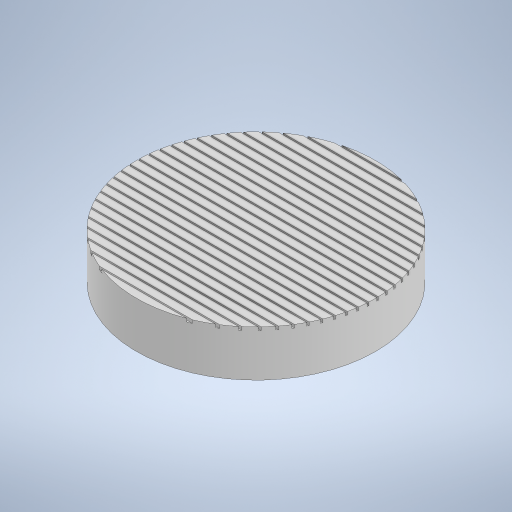
# Autodesk Inventor part: CircularTeflonHolder
Saved by Autodesk Inventor 2024 (Build 280153000, 153)
## iProperties
Created: 2023-08-11
Part Number: CircularTeflonHolder
Material: Generic
Document SubType Name: Modeling
Designer: Edwin
Density: 1 g/cm^3
Appearance: Default
Author: Edwin
Autodesk Inventor part; units mm, degrees
ref_plane "YZ Plane" through (0, 0, 0) normal (1, 0, 0) x (0, 1, 0)
ref_plane "XZ Plane" through (0, 0, 0) normal (0, 1, 0) x (-1, 0, 0)
ref_plane "XY Plane" through (0, 0, 0) normal (0, 0, 1) x (1, 0, 0)
sketch "Sketch1" plane through (0, 0, 0) normal (0, 1, 0) x (-1, 0, 0)
  circle A0 centre (0, 0) radius 38.1
  dimension "d0" = 76.2
  constraints: 1 centre point, 1 coincident
  measures "d0" diameter of A0
extrude "Extrusion1" add sketch "Sketch1" along normal blind 12.7
sketch "Sketch2" plane through (0, 0, 0) normal (0, -1, 0) x (1, 0, 0)
  circle A0 centre (0, 0) radius 38.1 projected
  circle A1 centre (0, 0) radius 32.1
  dimension "d3" = 6
  constraints: 1 centre point, 1 coincident
  measures "d3" radial gap between concentric circles of A0 A1
extrude "Extrusion2" add sketch "Sketch2" along normal blind 2
sketch "Sketch3" plane through (0, 0, 0) normal (1, 0, 0) x (0, 1, 0)
  line L0 (12.7, -38.1) -> (12.7, 38.1) projected
  line L1 (12.7, 38.1) -> (11.7, 38.1)
  line L2 (11.7, 38.1) -> (11.7, 38.6)
  line L3 (11.7, 38.6) -> (12.7, 38.6)
  line L4 (12.7, 38.6) -> (12.7, 38.1)
  line L5 (12.7, 35.1) -> (11.7, 35.1)
  line L6 (11.7, 35.1) -> (11.7, 35.6)
  line L7 (11.7, 35.6) -> (12.7, 35.6)
  line L8 (12.7, 35.6) -> (12.7, 35.1)
  line L9 (12.7, 32.1) -> (11.7, 32.1)
  line L10 (11.7, 32.1) -> (11.7, 32.6)
  line L11 (11.7, 32.6) -> (12.7, 32.6)
  line L12 (12.7, 32.6) -> (12.7, 32.1)
  line L13 (12.7, 29.1) -> (11.7, 29.1)
  line L14 (11.7, 29.1) -> (11.7, 29.6)
  line L15 (11.7, 29.6) -> (12.7, 29.6)
  line L16 (12.7, 29.6) -> (12.7, 29.1)
  line L17 (12.7, 26.1) -> (11.7, 26.1)
  line L18 (11.7, 26.1) -> (11.7, 26.6)
  line L19 (11.7, 26.6) -> (12.7, 26.6)
  line L20 (12.7, 26.6) -> (12.7, 26.1)
  line L21 (12.7, 23.1) -> (11.7, 23.1)
  line L22 (11.7, 23.1) -> (11.7, 23.6)
  line L23 (11.7, 23.6) -> (12.7, 23.6)
  line L24 (12.7, 23.6) -> (12.7, 23.1)
  line L25 (12.7, 20.1) -> (11.7, 20.1)
  line L26 (11.7, 20.1) -> (11.7, 20.6)
  line L27 (11.7, 20.6) -> (12.7, 20.6)
  line L28 (12.7, 20.6) -> (12.7, 20.1)
  line L29 (12.7, 17.1) -> (11.7, 17.1)
  line L30 (11.7, 17.1) -> (11.7, 17.6)
  line L31 (11.7, 17.6) -> (12.7, 17.6)
  line L32 (12.7, 17.6) -> (12.7, 17.1)
  line L33 (12.7, 14.1) -> (11.7, 14.1)
  line L34 (11.7, 14.1) -> (11.7, 14.6)
  line L35 (11.7, 14.6) -> (12.7, 14.6)
  line L36 (12.7, 14.6) -> (12.7, 14.1)
  line L37 (12.7, 11.1) -> (11.7, 11.1)
  line L38 (11.7, 11.1) -> (11.7, 11.6)
  line L39 (11.7, 11.6) -> (12.7, 11.6)
  line L40 (12.7, 11.6) -> (12.7, 11.1)
  line L41 (12.7, 8.1) -> (11.7, 8.1)
  line L42 (11.7, 8.1) -> (11.7, 8.6)
  line L43 (11.7, 8.6) -> (12.7, 8.6)
  line L44 (12.7, 8.6) -> (12.7, 8.1)
  line L45 (12.7, 5.1) -> (11.7, 5.1)
  line L46 (11.7, 5.1) -> (11.7, 5.6)
  line L47 (11.7, 5.6) -> (12.7, 5.6)
  line L48 (12.7, 5.6) -> (12.7, 5.1)
  line L49 (12.7, 2.1) -> (11.7, 2.1)
  line L50 (11.7, 2.1) -> (11.7, 2.6)
  line L51 (11.7, 2.6) -> (12.7, 2.6)
  line L52 (12.7, 2.6) -> (12.7, 2.1)
  line L53 (12.7, -0.9) -> (11.7, -0.9)
  line L54 (11.7, -0.9) -> (11.7, -0.4)
  line L55 (11.7, -0.4) -> (12.7, -0.4)
  line L56 (12.7, -0.4) -> (12.7, -0.9)
  line L57 (12.7, -3.9) -> (11.7, -3.9)
  line L58 (11.7, -3.9) -> (11.7, -3.4)
  line L59 (11.7, -3.4) -> (12.7, -3.4)
  line L60 (12.7, -3.4) -> (12.7, -3.9)
  line L61 (12.7, -6.9) -> (11.7, -6.9)
  line L62 (11.7, -6.9) -> (11.7, -6.4)
  line L63 (11.7, -6.4) -> (12.7, -6.4)
  line L64 (12.7, -6.4) -> (12.7, -6.9)
  line L65 (12.7, -9.9) -> (11.7, -9.9)
  line L66 (11.7, -9.9) -> (11.7, -9.4)
  line L67 (11.7, -9.4) -> (12.7, -9.4)
  line L68 (12.7, -9.4) -> (12.7, -9.9)
  line L69 (12.7, -12.9) -> (11.7, -12.9)
  line L70 (11.7, -12.9) -> (11.7, -12.4)
  line L71 (11.7, -12.4) -> (12.7, -12.4)
  line L72 (12.7, -12.4) -> (12.7, -12.9)
  line L73 (12.7, -15.9) -> (11.7, -15.9)
  line L74 (11.7, -15.9) -> (11.7, -15.4)
  line L75 (11.7, -15.4) -> (12.7, -15.4)
  line L76 (12.7, -15.4) -> (12.7, -15.9)
  line L77 (12.7, -18.9) -> (11.7, -18.9)
  line L78 (11.7, -18.9) -> (11.7, -18.4)
  line L79 (11.7, -18.4) -> (12.7, -18.4)
  line L80 (12.7, -18.4) -> (12.7, -18.9)
  line L81 (12.7, -21.9) -> (11.7, -21.9)
  line L82 (11.7, -21.9) -> (11.7, -21.4)
  line L83 (11.7, -21.4) -> (12.7, -21.4)
  line L84 (12.7, -21.4) -> (12.7, -21.9)
  line L85 (12.7, -24.9) -> (11.7, -24.9)
  line L86 (11.7, -24.9) -> (11.7, -24.4)
  line L87 (11.7, -24.4) -> (12.7, -24.4)
  line L88 (12.7, -24.4) -> (12.7, -24.9)
  line L89 (12.7, -27.9) -> (11.7, -27.9)
  line L90 (11.7, -27.9) -> (11.7, -27.4)
  line L91 (11.7, -27.4) -> (12.7, -27.4)
  line L92 (12.7, -27.4) -> (12.7, -27.9)
  line L93 (12.7, -30.9) -> (11.7, -30.9)
  line L94 (11.7, -30.9) -> (11.7, -30.4)
  line L95 (11.7, -30.4) -> (12.7, -30.4)
  line L96 (12.7, -30.4) -> (12.7, -30.9)
  line L97 (12.7, -33.9) -> (11.7, -33.9)
  line L98 (11.7, -33.9) -> (11.7, -33.4)
  line L99 (11.7, -33.4) -> (12.7, -33.4)
  line L100 (12.7, -33.4) -> (12.7, -33.9)
  line L101 (12.7, -36.9) -> (11.7, -36.9)
  line L102 (11.7, -36.9) -> (11.7, -36.4)
  line L103 (11.7, -36.4) -> (12.7, -36.4)
  line L104 (12.7, -36.4) -> (12.7, -36.9)
  line L105 (12.7, -39.9) -> (11.7, -39.9)
  line L106 (11.7, -39.9) -> (11.7, -39.4)
  line L107 (11.7, -39.4) -> (12.7, -39.4)
  line L108 (12.7, -39.4) -> (12.7, -39.9)
  line L109 (12.7, -42.9) -> (11.7, -42.9)
  line L110 (11.7, -42.9) -> (11.7, -42.4)
  line L111 (11.7, -42.4) -> (12.7, -42.4)
  line L112 (12.7, -42.4) -> (12.7, -42.9)
  line L113 (12.7, -45.9) -> (11.7, -45.9)
  line L114 (11.7, -45.9) -> (11.7, -45.4)
  line L115 (11.7, -45.4) -> (12.7, -45.4)
  line L116 (12.7, -45.4) -> (12.7, -45.9)
  point P0 (0, 0)
  point P1 (15, -89)
  point P2 (15, -88.5)
  point P3 (12.7, 35.6)
  point P4 (15, -82)
  point P5 (15, -81.5)
  point P6 (12.7, 32.6)
  point P7 (12.7, 29.6)
  point P8 (12.7, 26.6)
  point P9 (12.7, -36.4)
  point P10 (12.7, -30.4)
  point P11 (12.7, 23.6)
  point P12 (12.7, -27.4)
  point P13 (12.7, -24.4)
  point P14 (12.7, 17.6)
  point P15 (12.7, -21.4)
  point P16 (12.7, 14.6)
  point P17 (12.7, -18.4)
  point P18 (12.7, -33.4)
  point P19 (12.7, 11.6)
  point P20 (12.7, -15.4)
  point P21 (12.7, 8.6)
  point P22 (12.7, -12.4)
  point P23 (12.7, 5.6)
  point P24 (12.7, -9.4)
  point P25 (12.7, 2.6)
  point P26 (12.7, -6.4)
  point P27 (12.7, -0.4)
  point P28 (12.7, -3.4)
  point P29 (12.7, 20.6)
  point P30 (15, -96)
  point P31 (15, -95.5)
  dimension "d6" = 1
  dimension "d7" = 0.5
  dimension "d10" = 3
  constraints: 232 end point, 112 vertical alignment, 58 parallel, 56 collinear, 1 horizontal, 1 perpendicular, 1 other
  measures "d6" distance of L2.end L3.end
  measures "d7" distance of L1.end L2.end
  measures "d10" distance of L2.end L6.end
extrude "Extrusion3" cut sketch "Sketch3" along normal mid plane 200
body "Solid1"
